Autodesk Fusion 360 part; units mm, degrees
(part 13 of 25)
  arc A2546 (13.97, 2.3813) -> (13.97, 2.6987) centre (13.97, 2.54) ccw
  arc A2547 (73.405, 4.2862) -> (73.405, 4.6038) centre (73.405, 4.445) ccw
  arc A2548 (40.64, 5.2388) -> (40.64, 4.9212) centre (40.64, 5.08) ccw
  arc A2549 (38.1, 5.2388) -> (38.1, 4.9212) centre (38.1, 5.08) ccw
  arc A2550 (41.9535, 4.9212) -> (41.9535, 5.2388) centre (41.9535, 5.08) ccw
  arc A2551 (3.9718, 4.9212) -> (3.9718, 5.2388) centre (3.9718, 5.08) ccw
  arc A2552 (34.3335, 4.9212) -> (34.3335, 5.2388) centre (34.3335, 5.08) ccw
  arc A2553 (31.7935, 4.9212) -> (31.7935, 5.2388) centre (31.7935, 5.08) ccw
  arc A2554 (39.8168, 4.9212) -> (39.8168, 5.2388) centre (39.8168, 5.08) ccw
  arc A2555 (82.5144, 3.3338) -> (82.5144, 3.0163) centre (82.5144, 3.1751) ccw
  line L888 (34.2465, 5.08) -> (34.3335, 5.08)
  line L889 (41.4632, 5.08) -> (41.9535, 5.08)
  arc A2556 (84.2253, 1.7463) -> (84.2253, 2.0638) centre (84.2253, 1.9051) ccw
  arc A2557 (5.8036, 2.6987) -> (5.8036, 2.3813) centre (5.8036, 2.54) ccw
  arc A2558 (15.0528, 5.2388) -> (15.0528, 4.9212) centre (15.0528, 5.08) ccw
  arc A2559 (80.0301, 1.1113) -> (80.0301, 1.4287) centre (80.0301, 1.27) ccw
  arc A2560 (13.97, 3.6513) -> (13.97, 3.9688) centre (13.97, 3.81) ccw
  arc A2561 (84.2253, 3.6513) -> (84.2253, 3.9688) centre (84.2253, 3.81) ccw
  arc A2562 (6.477, 3.9688) -> (6.477, 3.6513) centre (6.477, 3.81) ccw
  arc A2563 (12.8872, 4.9212) -> (12.8872, 5.2388) centre (12.8872, 5.08) ccw
  arc A2564 (13.97, 2.6987) -> (13.97, 2.3813) centre (13.97, 2.54) ccw
  arc A2565 (37.2768, 4.9212) -> (37.2768, 5.2388) centre (37.2768, 5.08) ccw
  arc A2566 (72.7411, 1.7463) -> (72.7411, 2.0638) centre (72.7411, 1.9051) ccw
  arc A2567 (32.964, 1.1113) -> (32.964, 1.4287) centre (32.964, 1.27) ccw
  arc A2568 (68.4207, 3.9688) -> (68.4207, 3.6513) centre (68.4207, 3.81) ccw
  arc A2569 (57.0166, 33.4949) -> (56.6991, 33.4949) centre (56.8578, 33.4949) ccw
  arc A2570 (84.2253, 3.0163) -> (84.2253, 3.3338) centre (84.2253, 3.1751) ccw
  arc A2571 (56.9702, 19.5673) -> (56.7456, 19.3428) centre (56.8579, 19.455) ccw
  arc A2572 (32.964, 2.3813) -> (32.964, 2.6987) centre (32.964, 2.54) ccw
  arc A2573 (56.7962, 33.6406) -> (57.0895, 33.5191) centre (56.9428, 33.5799) ccw
  arc A2574 (40.64, 5.8738) -> (40.64, 5.5562) centre (40.64, 5.715) ccw
  arc A2575 (62.1865, 5.2388) -> (62.1865, 4.9212) centre (62.1865, 5.08) ccw
  line L890 (54.5665, 5.08) -> (54.6535, 5.08)
  arc A2576 (3.4036, 6.1913) -> (3.4036, 6.5088) centre (3.4036, 6.3501) ccw
  arc A2577 (0.7747, 4.6038) -> (0.7747, 4.2862) centre (0.7747, 4.445) ccw
  arc A2578 (6.731, 6.5088) -> (6.731, 6.1913) centre (6.731, 6.3501) ccw
  arc A2579 (68.5588, 3.3338) -> (68.5588, 3.0163) centre (68.5588, 3.1751) ccw
  arc A2580 (82.2759, 3.9688) -> (82.2759, 3.6513) centre (82.2759, 3.81) ccw
  arc A2581 (52.0265, 5.2388) -> (52.0265, 4.9212) centre (52.0265, 5.08) ccw
  arc A2582 (38.9232, 5.2388) -> (38.9232, 4.9212) centre (38.9232, 5.08) ccw
  arc A2583 (62.2735, 4.9212) -> (62.2735, 5.2388) centre (62.2735, 5.08) ccw
  line L891 (59.6465, 5.08) -> (59.7335, 5.08)
  line L892 (46.9465, 5.08) -> (47.0335, 5.08)
  arc A2584 (84.2253, 4.9212) -> (84.2253, 5.2388) centre (84.2253, 5.08) ccw
  arc A2585 (36.7865, 5.2388) -> (36.7865, 4.9212) centre (36.7865, 5.08) ccw
  line L893 (38.9232, 5.08) -> (39.8168, 5.08)
  line L894 (64.7265, 5.08) -> (64.8135, 5.08)
  line L895 (67.2665, 5.08) -> (67.3535, 5.08)
  arc A2586 (15.6337, 5.8738) -> (15.6337, 5.5562) centre (15.6337, 5.715) ccw
  arc A2587 (40.64, 5.5562) -> (40.64, 5.8738) centre (40.64, 5.715) ccw
  arc A2588 (74.7818, 5.8738) -> (74.7818, 5.5562) centre (74.7818, 5.715) ccw
  arc A2589 (3.4036, 5.5562) -> (3.4036, 5.8738) centre (3.4036, 5.715) ccw
  arc A2590 (67.3535, 4.9212) -> (67.3535, 5.2388) centre (67.3535, 5.08) ccw
  arc A2591 (52.1135, 4.9212) -> (52.1135, 5.2388) centre (52.1135, 5.08) ccw
  arc A2592 (54.6535, 4.9212) -> (54.6535, 5.2388) centre (54.6535, 5.08) ccw
  arc A2593 (12.6114, 4.2862) -> (12.6114, 4.6038) centre (12.6114, 4.445) ccw
  arc A2594 (15.3286, 4.6038) -> (15.3286, 4.2862) centre (15.3286, 4.445) ccw
  arc A2595 (38.1, 4.9212) -> (38.1, 5.2388) centre (38.1, 5.08) ccw
  arc A2596 (64.7265, 5.2388) -> (64.7265, 4.9212) centre (64.7265, 5.08) ccw
  arc A2597 (32.964, 3.0163) -> (32.964, 3.3338) centre (32.964, 3.1751) ccw
  arc A2598 (0.7747, 5.2388) -> (0.7747, 4.9212) centre (0.7747, 5.08) ccw
  arc A2599 (79.9074, 4.2862) -> (79.9074, 4.6038) centre (79.9074, 4.445) ccw
  arc A2600 (44.4065, 5.2388) -> (44.4065, 4.9212) centre (44.4065, 5.08) ccw
  arc A2601 (57.1065, 5.2388) -> (57.1065, 4.9212) centre (57.1065, 5.08) ccw
  arc A2602 (12.3063, 5.5562) -> (12.3063, 5.8738) centre (12.3063, 5.715) ccw
  arc A2603 (3.7214, 4.2862) -> (3.7214, 4.6038) centre (3.7214, 4.445) ccw
  arc A2604 (64.8135, 4.9212) -> (64.8135, 5.2388) centre (64.8135, 5.08) ccw
  arc A2605 (84.2253, 5.5562) -> (84.2253, 5.8738) centre (84.2253, 5.715) ccw
  arc A2606 (34.2465, 5.2388) -> (34.2465, 4.9212) centre (34.2465, 5.08) ccw
  arc A2607 (44.4935, 4.9212) -> (44.4935, 5.2388) centre (44.4935, 5.08) ccw
  line L896 (36.7865, 5.08) -> (37.2768, 5.08)
  arc A2608 (73.7116, 5.5562) -> (73.7116, 5.8738) centre (73.7116, 5.715) ccw
  arc A2609 (84.2253, 4.2862) -> (84.2253, 4.6038) centre (84.2253, 4.445) ccw
  arc A2610 (0.7747, 3.9688) -> (0.7747, 3.6513) centre (0.7747, 3.81) ccw
  arc A2611 (3.6576, 3.6513) -> (3.6576, 3.9688) centre (3.6576, 3.81) ccw
  arc A2612 (49.4865, 5.2388) -> (49.4865, 4.9212) centre (49.4865, 5.08) ccw
  arc A2613 (75.0884, 4.6038) -> (75.0884, 4.2862) centre (75.0884, 4.445) ccw
  arc A2614 (59.7335, 4.9212) -> (59.7335, 5.2388) centre (59.7335, 5.08) ccw
  arc A2615 (69.8065, 5.2388) -> (69.8065, 4.9212) centre (69.8065, 5.08) ccw
  arc A2616 (6.1628, 5.2388) -> (6.1628, 4.9212) centre (6.1628, 5.08) ccw
  arc A2617 (81.5908, 4.6038) -> (81.5908, 4.2862) centre (81.5908, 4.445) ccw
  arc A2618 (29.4986, 5.5562) -> (29.4986, 5.8738) centre (29.4986, 5.715) ccw
  arc A2619 (38.1, 5.8738) -> (38.1, 5.5562) centre (38.1, 5.715) ccw
  arc A2620 (44.4935, 7.4612) -> (44.4935, 7.7788) centre (44.4935, 7.62) ccw
  arc A2621 (40.64, 6.8262) -> (40.64, 7.1438) centre (40.64, 6.985) ccw
  arc A2622 (82.1916, 6.5088) -> (82.1916, 6.1913) centre (82.1916, 6.3501) ccw
  arc A2623 (57.1935, 4.9212) -> (57.1935, 5.2388) centre (57.1935, 5.08) ccw
  arc A2624 (80.214, 5.5562) -> (80.214, 5.8738) centre (80.214, 5.715) ccw
  arc A2625 (31.7935, 7.4612) -> (31.7935, 7.7788) centre (31.7935, 7.62) ccw
  arc A2626 (34.2465, 7.7788) -> (34.2465, 7.4612) centre (34.2465, 7.62) ccw
  arc A2627 (46.9465, 5.2388) -> (46.9465, 4.9212) centre (46.9465, 5.08) ccw
  arc A2628 (41.4632, 7.7788) -> (41.4632, 7.4612) centre (41.4632, 7.62) ccw
  arc A2629 (54.5665, 5.2388) -> (54.5665, 4.9212) centre (54.5665, 5.08) ccw
  arc A2630 (3.9972, 7.4612) -> (3.9972, 7.7788) centre (3.9972, 7.62) ccw
  arc A2631 (40.64, 7.1438) -> (40.64, 6.8262) centre (40.64, 6.985) ccw
  arc A2632 (12.3063, 6.1913) -> (12.3063, 6.5088) centre (12.3063, 6.3501) ccw
  arc A2633 (15.6337, 6.5088) -> (15.6337, 6.1913) centre (15.6337, 6.3501) ccw
  arc A2634 (49.5735, 4.9212) -> (49.5735, 5.2388) centre (49.5735, 5.08) ccw
  arc A2635 (70.7429, 6.8262) -> (70.7429, 7.1438) centre (70.7429, 6.985) ccw
  arc A2636 (0.7747, 7.7788) -> (0.7747, 7.4612) centre (0.7747, 7.62) ccw
  line L897 (57.1065, 5.08) -> (57.1935, 5.08)
  line L898 (62.1865, 5.08) -> (62.2735, 5.08)
  arc A2637 (0.7747, 6.5088) -> (0.7747, 6.1913) centre (0.7747, 6.3501) ccw
  arc A2638 (67.2665, 5.2388) -> (67.2665, 4.9212) centre (67.2665, 5.08) ccw
  arc A2639 (38.1, 7.7788) -> (38.1, 7.4612) centre (38.1, 7.62) ccw
  arc A2640 (70.2277, 7.1438) -> (70.2277, 6.8262) centre (70.2277, 6.985) ccw
  arc A2641 (34.3335, 7.4612) -> (34.3335, 7.7788) centre (34.3335, 7.62) ccw
  arc A2642 (79.3067, 6.1913) -> (79.3067, 6.5088) centre (79.3067, 6.3501) ccw
  line L899 (38.1, 6.35) -> (40.64, 6.35)
  arc A2643 (15.6337, 7.1438) -> (15.6337, 6.8262) centre (15.6337, 6.985) ccw
  arc A2644 (38.1, 5.5562) -> (38.1, 5.8738) centre (38.1, 5.715) ccw
  arc A2645 (0.7747, 5.8738) -> (0.7747, 5.5562) centre (0.7747, 5.715) ccw
  arc A2646 (59.6465, 5.2388) -> (59.6465, 4.9212) centre (59.6465, 5.08) ccw
  arc A2647 (75.6891, 6.5088) -> (75.6891, 6.1913) centre (75.6891, 6.3501) ccw
  arc A2648 (40.64, 7.7788) -> (40.64, 7.4612) centre (40.64, 7.62) ccw
  arc A2649 (6.731, 5.8738) -> (6.731, 5.5562) centre (6.731, 5.715) ccw
  line L900 (46.9465, 7.62) -> (47.0335, 7.62)
  arc A2650 (40.64, 6.1913) -> (40.64, 6.5088) centre (40.64, 6.3501) ccw
  arc A2651 (47.0335, 7.4612) -> (47.0335, 7.7788) centre (47.0335, 7.62) ccw
  arc A2652 (6.1374, 7.7788) -> (6.1374, 7.4612) centre (6.1374, 7.62) ccw
  arc A2653 (3.4036, 6.8262) -> (3.4036, 7.1438) centre (3.4036, 6.985) ccw
  arc A2654 (38.1, 6.8262) -> (38.1, 7.1438) centre (38.1, 6.985) ccw
  arc A2655 (0.7747, 7.1438) -> (0.7747, 6.8262) centre (0.7747, 6.985) ccw
  arc A2656 (11.317, 7.4612) -> (11.317, 7.7788) centre (11.317, 7.62) ccw
  arc A2657 (81.2842, 5.8738) -> (81.2842, 5.5562) centre (81.2842, 5.715) ccw
  arc A2658 (28.8636, 6.1913) -> (28.8636, 6.5088) centre (28.8636, 6.3501) ccw
  arc A2659 (70.2277, 5.8738) -> (70.2277, 5.5562) centre (70.2277, 5.715) ccw
  line L901 (44.4065, 5.08) -> (44.4935, 5.08)
  arc A2660 (38.1, 7.1438) -> (38.1, 6.8262) centre (38.1, 6.985) ccw
  arc A2661 (41.9535, 7.4612) -> (41.9535, 7.7788) centre (41.9535, 7.62) ccw
  line L902 (49.4865, 5.08) -> (49.5735, 5.08)
  arc A2662 (47.0335, 4.9212) -> (47.0335, 5.2388) centre (47.0335, 5.08) ccw
  line L903 (52.0265, 5.08) -> (52.1135, 5.08)
  arc A2663 (11.952, 6.8262) -> (11.952, 7.1438) centre (11.952, 6.985) ccw
  arc A2664 (59.6465, 7.7788) -> (59.6465, 7.4612) centre (59.6465, 7.62) ccw
  arc A2665 (84.2253, 8.0963) -> (84.2253, 8.4138) centre (84.2253, 8.2551) ccw
  arc A2666 (54.6535, 7.4612) -> (54.6535, 7.7788) centre (54.6535, 7.62) ccw
  arc A2667 (40.64, 7.4612) -> (40.64, 7.7788) centre (40.64, 7.62) ccw
  line L904 (49.4865, 7.62) -> (49.5735, 7.62)
  line L905 (62.1865, 7.62) -> (62.2735, 7.62)
  arc A2668 (26.3236, 8.7313) -> (26.3236, 9.0488) centre (26.3236, 8.89) ccw
  arc A2669 (82.983, 8.4138) -> (82.983, 8.0963) centre (82.983, 8.2551) ccw
  arc A2670 (37.2768, 7.4612) -> (37.2768, 7.7788) centre (37.2768, 7.62) ccw
  line L906 (34.2465, 7.62) -> (34.3335, 7.62)
  arc A2671 (44.4065, 7.7788) -> (44.4065, 7.4612) centre (44.4065, 7.62) ccw
  arc A2672 (30.8264, 7.7788) -> (30.8264, 7.4612) centre (30.8264, 7.62) ccw
  arc A2673 (84.2253, 6.8262) -> (84.2253, 7.1438) centre (84.2253, 6.985) ccw
  arc A2674 (72.8043, 6.1913) -> (72.8043, 6.5088) centre (72.8043, 6.3501) ccw
  arc A2675 (54.5665, 7.7788) -> (54.5665, 7.4612) centre (54.5665, 7.62) ccw
  arc A2676 (15.0528, 7.7788) -> (15.0528, 7.4612) centre (15.0528, 7.62) ccw
  arc A2677 (27.5936, 7.4612) -> (27.5936, 7.7788) centre (27.5936, 7.62) ccw
  arc A2678 (44.7421, 8.0963) -> (44.7421, 8.4138) centre (44.7421, 8.2551) ccw
  arc A2679 (38.1, 7.4612) -> (38.1, 7.7788) centre (38.1, 7.62) ccw
  arc A2680 (39.8168, 7.4612) -> (39.8168, 7.7788) centre (39.8168, 7.62) ccw
  arc A2681 (52.1135, 7.4612) -> (52.1135, 7.7788) centre (52.1135, 7.62) ccw
  line L907 (69.8065, 7.62) -> (70.1079, 7.62)
  arc A2682 (26.9586, 8.0963) -> (26.9586, 8.4138) centre (26.9586, 8.2551) ccw
  arc A2683 (28.2286, 6.8262) -> (28.2286, 7.1438) centre (28.2286, 6.985) ccw
  arc A2684 (84.2253, 6.1913) -> (84.2253, 6.5088) centre (84.2253, 6.3501) ccw
  arc A2685 (82.4863, 7.1438) -> (82.4863, 6.8262) centre (82.4863, 6.985) ccw
  arc A2686 (13.448, 8.4138) -> (13.448, 8.0963) centre (13.448, 8.2551) ccw
  arc A2687 (70.3453, 6.5088) -> (70.3453, 6.1913) centre (70.3453, 6.3501) ccw
  arc A2688 (46.9465, 7.7788) -> (46.9465, 7.4612) centre (46.9465, 7.62) ccw
  arc A2689 (29.5564, 9.0488) -> (29.5564, 8.7313) centre (29.5564, 8.89) ccw
  arc A2690 (46.6979, 8.4138) -> (46.6979, 8.0963) centre (46.6979, 8.2551) ccw
  arc A2691 (38.1, 6.5088) -> (38.1, 6.1913) centre (38.1, 6.3501) ccw
  arc A2692 (52.0265, 7.7788) -> (52.0265, 7.4612) centre (52.0265, 7.62) ccw
  line L908 (57.1065, 7.62) -> (57.1935, 7.62)
  arc A2693 (59.7335, 7.4612) -> (59.7335, 7.7788) centre (59.7335, 7.62) ccw
  line L909 (64.7265, 7.62) -> (64.8135, 7.62)
  arc A2694 (38.9232, 7.7788) -> (38.9232, 7.4612) centre (38.9232, 7.62) ccw
  arc A2695 (67.2665, 7.7788) -> (67.2665, 7.4612) centre (67.2665, 7.62) ccw
  arc A2696 (69.4729, 8.0963) -> (69.4729, 8.4138) centre (69.4729, 8.2551) ccw
  arc A2697 (36.7865, 7.7788) -> (36.7865, 7.4612) centre (36.7865, 7.62) ccw
  arc A2698 (46.6979, 9.0488) -> (46.6979, 8.7313) centre (46.6979, 8.89) ccw
  arc A2699 (6.731, 7.1438) -> (6.731, 6.8262) centre (6.731, 6.985) ccw
  arc A2700 (68.8379, 8.7313) -> (68.8379, 9.0488) centre (68.8379, 8.89) ccw
  arc A2701 (82.5144, 7.7788) -> (82.5144, 7.4612) centre (82.5144, 7.62) ccw
  arc A2702 (64.8135, 7.4612) -> (64.8135, 7.7788) centre (64.8135, 7.62) ccw
  line L910 (59.6465, 7.62) -> (59.7335, 7.62)
  arc A2703 (4.1275, 8.7313) -> (4.1275, 9.0488) centre (4.1275, 8.89) ccw
  line L911 (52.0265, 7.62) -> (52.1135, 7.62)
  arc A2704 (84.2253, 8.7313) -> (84.2253, 9.0488) centre (84.2253, 8.89) ccw
  arc A2705 (0.7747, 10.3187) -> (0.7747, 10.0013) centre (0.7747, 10.16) ccw
  arc A2706 (30.1914, 8.4138) -> (30.1914, 8.0963) centre (30.1914, 8.2551) ccw
  arc A2707 (28.2864, 10.3187) -> (28.2864, 10.0013) centre (28.2864, 10.16) ccw
  arc A2708 (10.4521, 8.7313) -> (10.4521, 9.0488) centre (10.4521, 8.89) ccw
  arc A2709 (67.3535, 7.4612) -> (67.3535, 7.7788) centre (67.3535, 7.62) ccw
  line L912 (54.5665, 7.62) -> (54.6535, 7.62)
  arc A2710 (64.7265, 7.7788) -> (64.7265, 7.4612) centre (64.7265, 7.62) ccw
  arc A2711 (79.7385, 8.7313) -> (79.7385, 9.0488) centre (79.7385, 8.89) ccw
  arc A2712 (57.1065, 7.7788) -> (57.1065, 7.4612) centre (57.1065, 7.62) ccw
  arc A2713 (3.6263, 10.6363) -> (3.6263, 10.9537) centre (3.6263, 10.795) ccw
  arc A2714 (14.4213, 10.0013) -> (14.4213, 10.3187) centre (14.4213, 10.16) ccw
  arc A2715 (12.813, 9.0488) -> (12.813, 8.7313) centre (12.813, 8.89) ccw
  arc A2716 (12.4079, 10.3187) -> (12.4079, 10.0013) centre (12.4079, 10.16) ccw
  arc A2717 (81.6991, 10.0013) -> (81.6991, 10.3187) centre (81.6991, 10.16) ccw
  arc A2718 (6.0833, 9.6837) -> (6.0833, 9.3663) centre (6.0833, 9.525) ccw
  arc A2719 (84.2253, 7.4612) -> (84.2253, 7.7788) centre (84.2253, 7.62) ccw
  arc A2720 (62.1865, 7.7788) -> (62.1865, 7.4612) centre (62.1865, 7.62) ccw
  arc A2721 (69.8065, 7.7788) -> (69.8065, 7.4612) centre (69.8065, 7.62) ccw
  arc A2722 (46.6979, 10.3187) -> (46.6979, 10.0013) centre (46.6979, 10.16) ccw
  arc A2723 (66.0563, 10.0013) -> (66.0563, 10.3187) centre (66.0563, 10.16) ccw
  arc A2724 (76.313, 10.3187) -> (76.313, 10.0013) centre (76.313, 10.16) ccw
  arc A2725 (6.0833, 9.0488) -> (6.0833, 8.7313) centre (6.0833, 8.89) ccw
  arc A2726 (84.2253, 10.0013) -> (84.2253, 10.3187) centre (84.2253, 10.16) ccw
  arc A2727 (70.372, 10.0013) -> (70.372, 10.3187) centre (70.372, 10.16) ccw
  arc A2728 (83.6549, 10.3187) -> (83.6549, 10.0013) centre (83.6549, 10.16) ccw
  arc A2729 (49.4865, 7.7788) -> (49.4865, 7.4612) centre (49.4865, 7.62) ccw
  arc A2730 (4.1275, 10.0013) -> (4.1275, 10.3187) centre (4.1275, 10.16) ccw
  arc A2731 (83.5524, 9.0488) -> (83.5524, 8.7313) centre (83.5524, 8.89) ccw
  arc A2732 (6.0833, 8.4138) -> (6.0833, 8.0963) centre (6.0833, 8.2551) ccw
  arc A2733 (71.007, 9.3663) -> (71.007, 9.6837) centre (71.007, 9.525) ccw
  arc A2734 (57.1935, 7.4612) -> (57.1935, 7.7788) centre (57.1935, 7.62) ccw
  arc A2735 (0.7747, 10.9537) -> (0.7747, 10.6363) centre (0.7747, 10.795) ccw
  arc A2736 (10.682, 8.0963) -> (10.682, 8.4138) centre (10.682, 8.2551) ccw
  arc A2737 (25.0536, 10.0013) -> (25.0536, 10.3187) centre (25.0536, 10.16) ccw
  arc A2738 (28.9214, 9.6837) -> (28.9214, 9.3663) centre (28.9214, 9.525) ccw
  arc A2739 (0.7747, 8.4138) -> (0.7747, 8.0963) centre (0.7747, 8.2551) ccw
  arc A2740 (44.7421, 8.7313) -> (44.7421, 9.0488) centre (44.7421, 8.89) ccw
  line L913 (67.2665, 7.62) -> (67.3535, 7.62)
  arc A2741 (4.1275, 8.0963) -> (4.1275, 8.4138) centre (4.1275, 8.2551) ccw
  arc A2742 (16.1095, 10.3187) -> (16.1095, 10.0013) centre (16.1095, 10.16) ccw
  arc A2743 (83.6549, 9.6837) -> (83.6549, 9.3663) centre (83.6549, 9.525) ccw
  arc A2744 (62.2735, 7.4612) -> (62.2735, 7.7788) centre (62.2735, 7.62) ccw
  arc A2745 (71.6038, 9.0488) -> (71.6038, 8.7313) centre (71.6038, 8.89) ccw
  arc A2746 (70.1079, 7.4612) -> (70.1079, 7.7788) centre (70.1079, 7.62) ccw
  arc A2747 (0.7747, 9.0488) -> (0.7747, 8.7313) centre (0.7747, 8.89) ccw
  arc A2748 (49.5735, 7.4612) -> (49.5735, 7.7788) centre (49.5735, 7.62) ccw
  arc A2749 (70.3338, 10.3187) -> (70.3338, 10.0013) centre (70.3338, 10.16) ccw
  arc A2750 (25.6886, 9.3663) -> (25.6886, 9.6837) centre (25.6886, 9.525) ccw
  line L914 (70.3338, 10.16) -> (70.372, 10.16)
  line L915 (70.9688, 9.525) -> (71.007, 9.525)
  arc A2751 (12.4079, 9.6837) -> (12.4079, 9.3663) centre (12.4079, 9.525) ccw
  arc A2752 (84.2253, 9.3663) -> (84.2253, 9.6837) centre (84.2253, 9.525) ccw
  arc A2753 (81.4871, 9.3663) -> (81.4871, 9.6837) centre (81.4871, 9.525) ccw
  arc A2754 (69.102, 11.2713) -> (69.102, 11.5887) centre (69.102, 11.43) ccw
  arc A2755 (81.5916, 11.2713) -> (81.5916, 11.5887) centre (81.5916, 11.43) ccw
  arc A2756 (13.7795, 11.2713) -> (13.7795, 11.5887) centre (13.7795, 11.43) ccw
  arc A2757 (6.0833, 10.3187) -> (6.0833, 10.0013) centre (6.0833, 10.16) ccw
  arc A2758 (0.7747, 9.6837) -> (0.7747, 9.3663) centre (0.7747, 9.525) ccw
  arc A2759 (0.7747, 11.5887) -> (0.7747, 11.2713) centre (0.7747, 11.43) ccw
  arc A2760 (44.7421, 10.6363) -> (44.7421, 10.9537) centre (44.7421, 10.795) ccw
  arc A2761 (77.583, 11.5887) -> (77.583, 11.2713) centre (77.583, 11.43) ccw
  arc A2762 (66.216, 9.3663) -> (66.216, 9.6837) centre (66.216, 9.525) ccw
  arc A2763 (70.9688, 9.6837) -> (70.9688, 9.3663) centre (70.9688, 9.525) ccw
  arc A2764 (16.8945, 11.5887) -> (16.8945, 11.2713) centre (16.8945, 11.43) ccw
  arc A2765 (27.0164, 11.5887) -> (27.0164, 11.2713) centre (27.0164, 11.43) ccw
  arc A2766 (84.2253, 11.2713) -> (84.2253, 11.5887) centre (84.2253, 11.43) ccw
  arc A2767 (44.7421, 10.0013) -> (44.7421, 10.3187) centre (44.7421, 10.16) ccw
  arc A2768 (10.4521, 10.0013) -> (10.4521, 10.3187) centre (10.4521, 10.16) ccw
  arc A2769 (13.8117, 11.9063) -> (13.8117, 12.2238) centre (13.8117, 12.0651) ccw
  arc A2770 (12.178, 12.2238) -> (12.178, 11.9063) centre (12.178, 12.0651) ccw
  arc A2771 (75.678, 9.6837) -> (75.678, 9.3663) centre (75.678, 9.525) ccw
  arc A2772 (10.4521, 9.3663) -> (10.4521, 9.6837) centre (10.4521, 9.525) ccw
  arc A2773 (76.948, 10.9537) -> (76.948, 10.6363) centre (76.948, 10.795) ccw
  arc A2774 (4.1275, 9.3663) -> (4.1275, 9.6837) centre (4.1275, 9.525) ccw
  arc A2775 (24.4185, 10.6363) -> (24.4185, 10.9537) centre (24.4185, 10.795) ccw
  arc A2776 (73.2432, 11.5887) -> (73.2432, 11.2713) centre (73.2432, 11.43) ccw
  arc A2777 (10.047, 11.2713) -> (10.047, 11.5887) centre (10.047, 11.43) ccw
  arc A2778 (13.7863, 10.6363) -> (13.7863, 10.9537) centre (13.7863, 10.795) ccw
  arc A2779 (23.7836, 11.2713) -> (23.7836, 11.5887) centre (23.7836, 11.43) ccw
  arc A2780 (84.2253, 10.6363) -> (84.2253, 10.9537) centre (84.2253, 10.795) ccw
  arc A2781 (73.2361, 8.7313) -> (73.2361, 9.0488) centre (73.2361, 8.89) ccw
  arc A2782 (66.216, 10.6363) -> (66.216, 10.9537) centre (66.216, 10.795) ccw
  arc A2783 (69.737, 10.6363) -> (69.737, 10.9537) centre (69.737, 10.795) ccw
  arc A2784 (3.6195, 11.2713) -> (3.6195, 11.5887) centre (3.6195, 11.43) ccw
  line L916 (69.6988, 10.795) -> (69.737, 10.795)
  arc A2785 (46.6979, 10.9537) -> (46.6979, 10.6363) centre (46.6979, 10.795) ccw
  arc A2786 (12.4079, 10.9537) -> (12.4079, 10.6363) centre (12.4079, 10.795) ccw
  arc A2787 (75.2573, 9.0488) -> (75.2573, 8.7313) centre (75.2573, 8.89) ccw
  arc A2788 (44.7421, 9.3663) -> (44.7421, 9.6837) centre (44.7421, 9.525) ccw
  arc A2789 (46.6979, 9.6837) -> (46.6979, 9.3663) centre (46.6979, 9.525) ccw
  arc A2790 (8.777, 12.5413) -> (8.777, 12.8588) centre (8.777, 12.7001) ccw
  arc A2791 (71.6638, 13.1763) -> (71.6638, 13.4938) centre (71.6638, 13.335) ccw
  arc A2792 (26.3814, 12.2238) -> (26.3814, 11.9063) centre (26.3814, 12.0651) ccw
  arc A2793 (44.7421, 11.2713) -> (44.7421, 11.5887) centre (44.7421, 11.43) ccw
  arc A2794 (27.6514, 10.9537) -> (27.6514, 10.6363) centre (27.6514, 10.795) ccw
  arc A2795 (72.517, 12.8588) -> (72.517, 12.5413) centre (72.517, 12.7001) ccw
  arc A2796 (23.1486, 11.9063) -> (23.1486, 12.2238) centre (23.1486, 12.0651) ccw
  arc A2797 (12.4079, 11.5887) -> (12.4079, 11.2713) centre (12.4079, 11.43) ccw
  arc A2798 (69.6988, 10.9537) -> (69.6988, 10.6363) centre (69.6988, 10.795) ccw
  arc A2799 (6.5845, 10.9537) -> (6.5845, 10.6363) centre (6.5845, 10.795) ccw
  arc A2800 (0.7747, 12.2238) -> (0.7747, 11.9063) centre (0.7747, 12.0651) ccw
  arc A2801 (72.517, 11.2713) -> (72.517, 11.5887) centre (72.517, 11.43) ccw
  arc A2802 (46.6979, 11.5887) -> (46.6979, 11.2713) centre (46.6979, 11.43) ccw
  arc A2803 (46.814, 13.4938) -> (46.814, 13.1763) centre (46.814, 13.335) ccw
  arc A2804 (84.1629, 12.2238) -> (84.1629, 11.9063) centre (84.1629, 12.0651) ccw
  arc A2805 (81.6991, 10.6363) -> (81.6991, 10.9537) centre (81.6991, 10.795) ccw
  arc A2806 (84.2253, 11.9063) -> (84.2253, 12.2238) centre (84.2253, 12.0651) ccw
  arc A2807 (83.7624, 11.5887) -> (83.7624, 11.2713) centre (83.7624, 11.43) ccw
  arc A2808 (16.7445, 10.9537) -> (16.7445, 10.6363) centre (16.7445, 10.795) ccw
  arc A2809 (0.7747, 12.8588) -> (0.7747, 12.5413) centre (0.7747, 12.7001) ccw
  arc A2810 (69.963, 13.4938) -> (69.963, 13.1763) centre (69.963, 13.335) ccw
  arc A2811 (6.5913, 11.5887) -> (6.5913, 11.2713) centre (6.5913, 11.43) ccw
  arc A2812 (72.517, 12.2238) -> (72.517, 11.9063) centre (72.517, 12.0651) ccw
  arc A2813 (10.4521, 10.6363) -> (10.4521, 10.9537) centre (10.4521, 10.795) ccw
  arc A2814 (9.412, 11.9063) -> (9.412, 12.2238) centre (9.412, 12.0651) ccw
  arc A2815 (15.5667, 13.1763) -> (15.5667, 13.4938) centre (15.5667, 13.335) ccw
  arc A2816 (78.218, 12.2238) -> (78.218, 11.9063) centre (78.218, 12.0651) ccw
  arc A2817 (22.5714, 12.2238) -> (22.5714, 11.9063) centre (22.5714, 12.0651) ccw
  arc A2818 (5.9241, 12.8588) -> (5.9241, 12.5413) centre (5.9241, 12.7001) ccw
  arc A2819 (68.467, 11.9063) -> (68.467, 12.2238) centre (68.467, 12.0651) ccw
  line L917 (71.233, 12.065) -> (71.2851, 12.065)
  arc A2820 (74.817, 11.2713) -> (74.817, 11.5887) centre (74.817, 11.43) ccw
  arc A2821 (25.1114, 13.4938) -> (25.1114, 13.1763) centre (25.1114, 13.335) ccw
  arc A2822 (6.5591, 12.2238) -> (6.5591, 11.9063) centre (6.5591, 12.0651) ccw
  arc A2823 (44.7421, 12.5413) -> (44.7421, 12.8588) centre (44.7421, 12.7001) ccw
  arc A2824 (72.517, 11.5887) -> (72.517, 11.2713) centre (72.517, 11.43) ccw
  arc A2825 (84.1629, 12.8588) -> (84.1629, 12.5413) centre (84.1629, 12.7001) ccw
  arc A2826 (44.626, 13.1763) -> (44.626, 13.4938) centre (44.626, 13.335) ccw
  arc A2827 (48.782, 13.1763) -> (48.782, 13.4938) centre (48.782, 13.335) ccw
  arc A2828 (0.7747, 13.4938) -> (0.7747, 13.1763) centre (0.7747, 13.335) ccw
  arc A2829 (10.908, 13.4938) -> (10.908, 13.1763) centre (10.908, 13.335) ccw
  arc A2830 (78.853, 12.8588) -> (78.853, 12.5413) centre (78.853, 12.7001) ccw
  arc A2831 (83.6549, 10.9537) -> (83.6549, 10.6363) centre (83.6549, 10.795) ccw
  arc A2832 (73.7489, 12.8588) -> (73.7489, 12.5413) centre (73.7489, 12.7001) ccw
  arc A2833 (3.6517, 11.9063) -> (3.6517, 12.2238) centre (3.6517, 12.0651) ccw
  arc A2834 (20.4787, 38.1) -> (20.1612, 38.1) centre (20.32, 38.1) ccw
  line L918 (20.32, 36.8681) -> (20.32, 38.1)
  arc A2835 (18.9206, 36.918) -> (19.1073, 37.1748) centre (19.014, 37.0464) ccw
  line L919 (20.32, 38.1) -> (20.32, 36.8681)
  arc A2836 (18.8322, 37.4097) -> (18.6077, 37.1852) centre (18.72, 37.2975) ccw
  arc A2837 (21.8762, 37.0319) -> (21.6896, 37.2888) centre (21.7829, 37.1604) ccw
  line L920 (18.518, 37.6271) -> (18.606, 37.4543)
  arc A2838 (21.5327, 37.1748) -> (21.7194, 36.918) centre (21.6261, 37.0464) ccw
  arc A2839 (21.0525, 37.0249) -> (21.1022, 36.7113) centre (21.0773, 36.8681) ccw
  line L921 (18.606, 37.4543) -> (18.72, 37.2975)
  arc A2840 (20.32, 38.2587) -> (20.32, 37.9412) centre (20.32, 38.0999) ccw
  arc A2841 (19.086, 37.1878) -> (18.9419, 36.9049) centre (19.014, 37.0464) ccw
  line L922 (20.32, 38.1) -> (18.4277, 38.1)
  arc A2842 (21.0774, 36.7094) -> (21.0774, 37.0268) centre (21.0774, 36.8681) ccw
  arc A2843 (18.7448, 37.0481) -> (18.9693, 37.2726) centre (18.8571, 37.1603) ccw
  arc A2844 (21.6981, 36.9049) -> (21.554, 37.1878) centre (21.6261, 37.0464) ccw
  arc A2845 (18.7344, 37.5477) -> (18.4776, 37.361) centre (18.606, 37.4543) ccw
  arc A2846 (21.3812, 37.0998) -> (21.5254, 36.8169) centre (21.4533, 36.9583) ccw
  line L923 (18.458, 37.8115) -> (18.518, 37.6271)
  arc A2847 (18.3012, 37.7867) -> (18.6148, 37.8364) centre (18.458, 37.8115) ccw
  line L924 (21.0774, 36.8681) -> (21.2689, 36.8984)
  arc A2848 (19.5378, 36.7113) -> (19.5875, 37.0249) centre (19.5627, 36.8681) ccw
  arc A2849 (18.367, 37.5781) -> (18.6689, 37.6762) centre (18.5179, 37.6272) ccw
  arc A2850 (18.6594, 37.6992) -> (18.3765, 37.555) centre (18.5179, 37.6271) ccw
  arc A2851 (20.1612, 38.1) -> (20.4787, 38.1) centre (20.32, 38.1) ccw
  arc A2852 (19.5626, 37.0268) -> (19.5626, 36.7094) centre (19.5626, 36.8681) ccw
  arc A2853 (18.269, 38.003) -> (18.5865, 38.003) centre (18.4277, 38.003) ccw
  arc A2854 (18.4277, 38.2588) -> (18.4277, 37.9413) centre (18.4277, 38.1) ccw
  line L925 (21.2689, 36.8984) -> (21.4533, 36.9584)
  line L926 (19.3711, 36.8984) -> (19.5626, 36.8681)
  arc A2855 (20.1612, 36.8681) -> (20.4787, 36.8681) centre (20.32, 36.8681) ccw
  arc A2856 (19.2358, 37.1093) -> (19.1377, 36.8074) centre (19.1867, 36.9583) ccw
  arc A2857 (18.5865, 38.1) -> (18.269, 38.1) centre (18.4277, 38.1) ccw
  arc A2858 (20.4787, 38.1) -> (20.1612, 38.1) centre (20.32, 38.1) ccw
  arc A2859 (19.1146, 36.8169) -> (19.2588, 37.0998) centre (19.1867, 36.9584) ccw
  arc A2860 (21.5406, 39.3753) -> (21.3965, 39.0924) centre (21.4686, 39.2339) ccw
  arc A2861 (20.32, 37.9413) -> (20.32, 38.2588) centre (20.32, 38.1) ccw
  arc A2862 (20.32, 37.9412) -> (20.32, 38.2587) centre (20.32, 38.0999) ccw
  line L927 (18.4277, 38.1) -> (18.4277, 38.003)
  arc A2863 (18.5845, 38.0279) -> (18.2709, 37.9782) centre (18.4277, 38.0031) ccw
  line L928 (20.32, 36.8681) -> (21.0774, 36.8681)
  arc A2864 (18.4277, 38.2587) -> (18.4277, 37.9412) centre (18.4277, 38.0999) ccw
  arc A2865 (21.5023, 36.8074) -> (21.4042, 37.1093) centre (21.4533, 36.9583) ccw
  line L929 (18.4277, 38.1) -> (20.32, 38.1)
  arc A2866 (18.9504, 37.2888) -> (18.7638, 37.0319) centre (18.8571, 37.1604) ccw
  arc A2867 (19.3221, 36.7475) -> (19.4202, 37.0494) centre (19.3712, 36.8984) ccw
  arc A2868 (20.32, 36.7093) -> (20.32, 37.0268) centre (20.32, 36.8681) ccw
  line L930 (19.1867, 36.9584) -> (19.3711, 36.8984)
  line L931 (19.5626, 36.8681) -> (20.32, 36.8681)
  arc A2869 (18.5915, 37.2042) -> (18.8484, 37.3908) centre (18.72, 37.2975) ccw
  arc A2870 (20.1613, 36.8681) -> (20.4788, 36.8681) centre (20.3201, 36.8681) ccw
  arc A2871 (20.4788, 38.1) -> (20.1613, 38.1) centre (20.3201, 38.1) ccw
  arc A2872 (21.2198, 37.0494) -> (21.3179, 36.7475) centre (21.2688, 36.8984) ccw
  line L932 (21.6261, 37.0464) -> (21.7829, 37.1604)
  line L933 (18.4277, 38.003) -> (18.458, 37.8115)
  arc A2873 (20.32, 37.9412) -> (20.32, 38.2587) centre (20.32, 38.0999) ccw
  line L934 (18.72, 37.2975) -> (18.8571, 37.1604)
  arc A2874 (18.4645, 37.3823) -> (18.7474, 37.5264) centre (18.6059, 37.4544) ccw
  arc A2875 (18.609, 37.8606) -> (18.3071, 37.7625) centre (18.4581, 37.8116) ccw
  arc A2876 (19.396, 37.0552) -> (19.3463, 36.7416) centre (19.3712, 36.8984) ccw
  line L935 (19.0139, 37.0464) -> (19.1867, 36.9584)
  line L936 (18.8571, 37.1604) -> (19.0139, 37.0464)
  arc A2877 (20.32, 37.0268) -> (20.32, 36.7094) centre (20.32, 36.8681) ccw
  arc A2878 (22.0252, 37.8364) -> (22.3388, 37.7867) centre (22.182, 37.8115) ccw
  arc A2879 (20.32, 38.2588) -> (20.32, 37.9413) centre (20.32, 38.1) ccw
  arc A2880 (21.554, 39.0122) -> (21.6981, 39.2951) centre (21.6261, 39.1536) ccw
  line L937 (21.8221, 39.3803) -> (22.1039, 39.6621)
  arc A2881 (22.031, 38.3394) -> (22.3329, 38.4375) centre (22.1819, 38.3884) ccw
  arc A2882 (22.0535, 38.1) -> (22.371, 38.1) centre (22.2123, 38.1) ccw
  arc A2883 (21.7194, 39.282) -> (21.5327, 39.0252) centre (21.626, 39.1536) ccw
  arc A2884 (21.4078, 39.3805) -> (21.5293, 39.0872) centre (21.4686, 39.2339) ccw
  line L938 (20.32, 38.1) -> (22.2123, 38.1)
  arc A2885 (22.3329, 37.7625) -> (22.031, 37.8606) centre (22.1819, 37.8116) ccw
  line L939 (22.2123, 38.1) -> (20.32, 38.1)
  arc A2886 (15.0857, 36.2682) -> (14.7923, 36.1467) centre (14.939, 36.2075) ccw
  arc A2887 (21.6896, 38.9112) -> (21.8762, 39.1681) centre (21.7829, 39.0397) ccw
  arc A2888 (22.3691, 37.9782) -> (22.0555, 38.0279) centre (22.2123, 38.0031) ccw
  line L940 (22.182, 37.8115) -> (22.2123, 38.003)
  line L941 (21.7829, 37.1604) -> (21.92, 37.2975)
  line L942 (22.2123, 38.197) -> (22.182, 38.3885)
  arc A2889 (20.4788, 38.1) -> (20.1613, 38.1) centre (20.3201, 38.1) ccw
  arc A2890 (22.0555, 38.1721) -> (22.3691, 38.2218) centre (22.2123, 38.197) ccw
  arc A2891 (25.5945, 39.5034) -> (25.5945, 39.8209) centre (25.5945, 39.6622) ccw
  line L943 (22.2123, 38.003) -> (22.2123, 38.1)
  line L944 (25.9539, 39.811) -> (26.5671, 40.4241)
  line L945 (22.2123, 38.1) -> (22.2123, 38.197)
  line L946 (21.6261, 39.1536) -> (21.4685, 39.2339)
  arc A2892 (25.5338, 39.8088) -> (25.6553, 39.5154) centre (25.5946, 39.6621) ccw
  arc A2893 (22.2123, 37.9412) -> (22.2123, 38.2587) centre (22.2123, 38.0999) ccw
  arc A2894 (22.0323, 37.1852) -> (21.8078, 37.4097) centre (21.92, 37.2975) ccw
  arc A2895 (20.1613, 38.1) -> (20.4788, 38.1) centre (20.3201, 38.1) ccw
  arc A2896 (22.2161, 39.5498) -> (21.9916, 39.7744) centre (22.1039, 39.6621) ccw
  line L947 (22.182, 38.3885) -> (22.122, 38.5729)
  line L948 (21.7829, 39.0396) -> (21.6261, 39.1536)
  line L949 (22.034, 37.4543) -> (22.122, 37.6271)
  line L950 (22.034, 38.7457) -> (21.92, 38.9025)
  arc A2897 (22.1039, 39.8209) -> (22.1039, 39.5034) centre (22.1039, 39.6622) ccw
  arc A2898 (21.8078, 38.7903) -> (22.0323, 39.0148) centre (21.92, 38.9026) ccw
  arc A2899 (21.8952, 39.1519) -> (21.6707, 38.9274) centre (21.783, 39.0396) ccw
  arc A2900 (22.2123, 37.9413) -> (22.2123, 38.2588) centre (22.2123, 38.1) ccw
  line L951 (21.92, 37.2975) -> (22.034, 37.4543)
  arc A2901 (22.0485, 38.9958) -> (21.7916, 38.8092) centre (21.92, 38.9025) ccw
  arc A2902 (21.7098, 39.4926) -> (21.9343, 39.2681) centre (21.822, 39.3803) ccw
  arc A2903 (22.1624, 37.361) -> (21.9056, 37.5477) centre (22.034, 37.4543) ccw
  arc A2904 (22.3388, 38.4133) -> (22.0252, 38.3636) centre (22.182, 38.3884) ccw
  arc A2905 (26.6793, 40.3118) -> (26.4548, 40.5364) centre (26.5671, 40.4241) ccw
  arc A2906 (21.6707, 37.2726) -> (21.8952, 37.0481) centre (21.783, 37.1603) ccw
  arc A2907 (22.371, 38.1) -> (22.0535, 38.1) centre (22.2123, 38.1) ccw
  line L952 (22.1039, 39.6621) -> (25.5945, 39.6621)
  line L953 (22.122, 37.6271) -> (22.182, 37.8115)
  arc A2908 (21.9056, 38.6523) -> (22.1624, 38.839) centre (22.034, 38.7457) ccw
  arc A2909 (21.8828, 39.2336) -> (21.7613, 39.527) centre (21.8221, 39.3803) ccw
  arc A2910 (21.9711, 37.6762) -> (22.273, 37.5781) centre (22.1221, 37.6272) ccw
  line L954 (25.5945, 39.6621) -> (25.9539, 39.811)
  arc A2911 (26.0147, 39.6643) -> (25.8932, 39.9576) centre (25.954, 39.8109) ccw
  arc A2912 (21.7916, 37.3908) -> (22.0485, 37.2042) centre (21.92, 37.2975) ccw
  line L955 (22.122, 38.5729) -> (22.034, 38.7457)
  line L956 (21.4685, 39.2339) -> (21.8221, 39.3803)
  arc A2913 (22.273, 38.6219) -> (21.9711, 38.5238) centre (22.1221, 38.5729) ccw
  arc A2914 (21.8926, 37.5264) -> (22.1755, 37.3823) centre (22.0341, 37.4544) ccw
  arc A2915 (20.32, 38.2587) -> (20.32, 37.9412) centre (20.32, 38.0999) ccw
  arc A2916 (22.2635, 37.555) -> (21.9806, 37.6992) centre (22.1221, 37.6271) ccw
  arc A2917 (22.0535, 38.003) -> (22.371, 38.003) centre (22.2123, 38.003) ccw
  arc A2918 (22.371, 38.197) -> (22.0535, 38.197) centre (22.2123, 38.197) ccw
  arc A2919 (22.1755, 38.8177) -> (21.8926, 38.6736) centre (22.0341, 38.7457) ccw
  arc A2920 (21.9806, 38.5008) -> (22.2635, 38.645) centre (22.1221, 38.5729) ccw
  line L957 (21.92, 38.9025) -> (21.7829, 39.0396)
  arc A2921 (37.4455, 43.2371) -> (37.4455, 43.5546) centre (37.4455, 43.3959) ccw
  arc A2922 (25.8417, 39.9232) -> (26.0662, 39.6987) centre (25.954, 39.811) ccw
  arc A2923 (38.1571, 41.2945) -> (38.4746, 41.2945) centre (38.3158, 41.2945) ccw
  arc A2924 (36.1023, 40.3118) -> (36.3268, 40.5364) centre (36.2145, 40.4241) ccw
  arc A2925 (27.1732, 40.5364) -> (27.3977, 40.3118) centre (27.2855, 40.4241) ccw
  arc A2926 (15.2717, 35.7874) -> (14.9542, 35.7874) centre (15.113, 35.7874) ccw
  arc A2927 (11.6574, 39.0842) -> (11.6574, 39.4017) centre (11.6574, 39.243) ccw
  arc A2928 (37.3332, 40.5364) -> (37.5577, 40.3118) centre (37.4455, 40.4241) ccw
  arc A2929 (36.2145, 43.5546) -> (36.2145, 43.2371) centre (36.2145, 43.3959) ccw
  arc A2930 (35.5029, 42.5255) -> (35.1854, 42.5255) centre (35.3441, 42.5255) ccw
  arc A2931 (12.2867, 38.6352) -> (12.5112, 38.8597) centre (12.399, 38.7475) ccw
  arc A2932 (4.3767, 40.6443) -> (4.1522, 40.4197) centre (4.2645, 40.532) ccw
  line L958 (15.113, 35.7874) -> (14.939, 36.2075)
  arc A2933 (14.7297, 36.6412) -> (14.5052, 36.4167) centre (14.6175, 36.529) ccw
  arc A2934 (14.5052, 36.4167) -> (14.7297, 36.6412) centre (14.6175, 36.529) ccw
  line L959 (37.4455, 40.4241) -> (38.3159, 41.2945)
  arc A2935 (15.5271, 34.9122) -> (15.2337, 34.7907) centre (15.3804, 34.8514) ccw
  arc A2936 (12.5112, 38.8597) -> (12.2867, 38.6352) centre (12.399, 38.7475) ccw
  line L960 (35.3441, 42.5255) -> (35.3441, 41.2945)
  arc A2937 (5.5534, 39.4017) -> (5.5534, 39.0842) centre (5.5534, 39.243) ccw
  arc A2938 (11.7181, 39.3897) -> (11.5966, 39.0963) centre (11.6573, 39.243) ccw
  line L961 (36.2145, 43.3959) -> (35.3441, 42.5255)
  arc A2939 (15.7924, 34.2399) -> (15.4749, 34.2399) centre (15.6337, 34.2399) ccw
  arc A2940 (35.2318, 42.6377) -> (35.4564, 42.4132) centre (35.3441, 42.5255) ccw
  line L962 (14.939, 36.2075) -> (14.6175, 36.529)
  line L963 (14.6175, 36.529) -> (12.399, 38.7475)
  line L964 (37.4455, 43.3959) -> (36.2145, 43.3959)
  line L965 (38.3159, 42.5255) -> (37.4455, 43.3959)
  arc A2941 (35.4564, 41.4068) -> (35.2318, 41.1823) centre (35.3441, 41.2946) ccw
  arc A2942 (28.2682, 41.1823) -> (28.0436, 41.4068) centre (28.1559, 41.2946) ccw
  line L966 (38.3159, 41.2945) -> (38.3159, 42.5255)
  arc A2943 (38.4282, 41.1823) -> (38.2036, 41.4068) centre (38.3159, 41.2945) ccw
  line L967 (12.399, 38.7475) -> (12.0775, 39.069)
  arc A2944 (14.8267, 36.0952) -> (15.0512, 36.3197) centre (14.939, 36.2075) ccw
  arc A2945 (27.2855, 40.2654) -> (27.2855, 40.5829) centre (27.2855, 40.4241) ccw
  line L968 (5.5534, 39.243) -> (4.2644, 40.532)
  arc A2946 (15.4749, 33.5781) -> (15.7924, 33.5781) centre (15.6337, 33.5781) ccw
  arc A2947 (15.487, 34.1792) -> (15.7804, 34.3007) centre (15.6337, 34.24) ccw
  line L969 (15.113, 35.1188) -> (15.113, 35.7874)
  line L970 (11.6574, 39.243) -> (5.5534, 39.243)
  arc A2948 (37.4455, 40.2654) -> (37.4455, 40.5829) centre (37.4455, 40.4241) ccw
  line L971 (12.0775, 39.069) -> (11.6574, 39.243)
  line L972 (15.3804, 34.8514) -> (15.113, 35.1188)
  arc A2949 (35.1854, 41.2945) -> (35.5029, 41.2945) centre (35.3441, 41.2945) ccw
  line L973 (15.6337, 33.5781) -> (15.6337, 34.2399)
  line L974 (27.2855, 40.4241) -> (28.1559, 41.2945)
  arc A2950 (38.4746, 42.5255) -> (38.1571, 42.5255) centre (38.3158, 42.5255) ccw
  arc A2951 (5.4412, 39.1307) -> (5.6657, 39.3553) centre (5.5535, 39.243) ccw
  line L975 (26.5671, 40.4241) -> (27.2855, 40.4241)
  line L976 (35.3441, 41.2945) -> (36.2145, 40.4241)
  arc A2952 (14.9663, 35.7266) -> (15.2597, 35.8481) centre (15.113, 35.7874) ccw
  line L977 (36.2145, 40.4241) -> (37.4455, 40.4241)
  arc A2953 (12.1897, 39.1812) -> (11.9652, 38.9567) centre (12.0775, 39.069) ccw
  arc A2954 (38.2036, 42.4132) -> (38.4282, 42.6377) centre (38.3159, 42.5255) ccw
  arc A2955 (12.0167, 38.9223) -> (12.1382, 39.2157) centre (12.0775, 39.069) ccw
  arc A2956 (26.5671, 40.5829) -> (26.5671, 40.2654) centre (26.5671, 40.4241) ccw
  arc A2957 (36.3268, 43.2836) -> (36.1023, 43.5082) centre (36.2145, 43.3959) ccw
  arc A2958 (36.2145, 40.5829) -> (36.2145, 40.2654) centre (36.2145, 40.4241) ccw
  arc A2959 (15.2253, 35.2311) -> (15.0007, 35.0066) centre (15.113, 35.1189) ccw
  line L978 (15.6337, 34.2399) -> (15.3804, 34.8514)
  arc A2960 (15.2682, 34.7392) -> (15.4927, 34.9637) centre (15.3805, 34.8514) ccw
  arc A2961 (37.5577, 43.5082) -> (37.3332, 43.2836) centre (37.4455, 43.3959) ccw
  arc A2962 (4.8214, 43.6691) -> (5.1147, 43.5476) centre (4.968, 43.6084) ccw
  arc A2963 (14.9542, 35.1188) -> (15.2717, 35.1188) centre (15.113, 35.1188) ccw
  line L979 (5.1943, 44.7456) -> (4.9681, 45.2917)
  line L980 (0.9017, 44.1544) -> (1.1279, 43.6083)
  arc A2964 (4.4378, 43.3026) -> (4.6623, 43.0781) centre (4.55, 43.1903) ccw
  arc A2965 (0.9812, 43.5476) -> (1.2746, 43.6691) centre (1.1279, 43.6084) ccw
  line L981 (5.1943, 42.2056) -> (4.9681, 42.7517)
  arc A2966 (1.0157, 45.4039) -> (1.2402, 45.1794) centre (1.128, 45.2917) ccw
  arc A2967 (0.755, 44.8063) -> (1.0484, 44.6848) centre (0.9017, 44.7456) ccw
  arc A2968 (4.2037, 40.6787) -> (4.3252, 40.3853) centre (4.2645, 40.532) ccw
  arc A2969 (5.341, 41.5537) -> (5.0476, 41.6752) centre (5.1943, 41.6145) ccw
  line L982 (4.9681, 42.7517) -> (4.5501, 43.1697)
  line L983 (1.5459, 45.7097) -> (1.1279, 45.2917)
  line L984 (1.5459, 43.1903) -> (1.5708, 43.18)
  arc A2970 (1.6582, 45.5974) -> (1.4336, 45.8219) centre (1.5459, 45.7097) ccw
  arc A2971 (4.0647, 46.0826) -> (3.9432, 45.7892) centre (4.004, 45.9359) ccw
  line L985 (4.9681, 45.2917) -> (4.5501, 45.7097)
  arc A2972 (1.2402, 43.7206) -> (1.0157, 43.496) centre (1.1279, 43.6083) ccw
  arc A2973 (0.7429, 44.1544) -> (1.0605, 44.1544) centre (0.9017, 44.1544) ccw
  arc A2974 (5.0803, 40.956) -> (4.8558, 41.1806) centre (4.9681, 41.0683) ccw
  line L986 (4.5501, 43.1903) -> (4.9681, 43.6083)
  line L987 (1.1279, 43.6083) -> (1.5459, 43.1903)
  line L988 (5.1943, 41.6144) -> (5.1943, 42.2056)
  arc A2975 (5.0355, 41.6144) -> (5.353, 41.6144) centre (5.1943, 41.6144) ccw
  arc A2976 (4.6108, 43.0436) -> (4.4894, 43.337) centre (4.5501, 43.1903) ccw
  line L989 (2.092, 45.9359) -> (1.5459, 45.7097)
  arc A2977 (5.341, 44.0937) -> (5.0476, 44.2152) centre (5.1943, 44.1544) ccw
  arc A2978 (4.4893, 45.563) -> (4.6108, 45.8563) centre (4.5501, 45.7097) ccw
  line L990 (4.5501, 43.1697) -> (4.5252, 43.18)
  arc A2979 (2.092, 46.0946) -> (2.092, 45.7771) centre (2.092, 45.9359) ccw
  line L991 (0.9017, 44.7456) -> (0.9017, 44.1544)
  line L992 (1.1279, 45.2917) -> (0.9017, 44.7456)
  arc A2980 (5.0355, 44.1544) -> (5.353, 44.1544) centre (5.1943, 44.1544) ccw
  arc A2981 (4.8558, 45.1794) -> (5.0803, 45.4039) centre (4.9681, 45.2917) ccw
  arc A2982 (4.4644, 43.3267) -> (4.5859, 43.0333) centre (4.5251, 43.18) ccw
  arc A2983 (1.4336, 43.0781) -> (1.6582, 43.3026) centre (1.5459, 43.1904) ccw
  arc A2984 (4.4893, 43.023) -> (4.6108, 43.3163) centre (4.55, 43.1696) ccw
  arc A2985 (1.0605, 44.7456) -> (0.7429, 44.7456) centre (0.9017, 44.7456) ccw
  line L993 (4.5501, 45.7097) -> (4.004, 45.9359)
  arc A2986 (5.353, 42.2056) -> (5.0355, 42.2056) centre (5.1943, 42.2056) ccw
  arc A2987 (1.0484, 44.2152) -> (0.755, 44.0937) centre (0.9017, 44.1544) ccw
  line L994 (4.9681, 41.0683) -> (5.1943, 41.6144)
  arc A2988 (5.1147, 42.8124) -> (4.8214, 42.6909) centre (4.9681, 42.7516) ccw
  arc A2989 (4.8558, 42.6394) -> (5.0803, 42.8639) centre (4.968, 42.7517) ccw
  line L995 (4.5252, 43.18) -> (4.5501, 43.1903)
  arc A2990 (5.0476, 44.6848) -> (5.341, 44.8063) centre (5.1943, 44.7456) ccw
  arc A2991 (4.5859, 43.3267) -> (4.4644, 43.0333) centre (4.5251, 43.18) ccw
  arc A2992 (5.1147, 45.3524) -> (4.8214, 45.2309) centre (4.968, 45.2916) ccw
  arc A2993 (2.1528, 45.7892) -> (2.0313, 46.0826) centre (2.0921, 45.9359) ccw
  arc A2994 (5.353, 44.7456) -> (5.0355, 44.7456) centre (5.1943, 44.7456) ccw
  arc A2995 (4.6108, 40.5036) -> (4.4893, 40.797) centre (4.5501, 40.6503) ccw
  arc A2996 (4.6623, 45.8219) -> (4.4378, 45.5974) centre (4.5501, 45.7097) ccw
  arc A2997 (5.0803, 43.496) -> (4.8558, 43.7206) centre (4.968, 43.6083) ccw
  arc A2998 (5.0476, 42.1448) -> (5.341, 42.2663) centre (5.1943, 42.2056) ccw
  line L996 (5.1943, 44.1544) -> (5.1943, 44.7456)
  arc A2999 (4.8214, 41.1291) -> (5.1147, 41.0076) centre (4.9681, 41.0684) ccw
  line L997 (4.2644, 40.532) -> (4.5501, 40.6503)
  line L998 (4.5501, 40.6503) -> (4.9681, 41.0683)
  arc A3000 (4.004, 45.7771) -> (4.004, 46.0946) centre (4.004, 45.9359) ccw
  arc A3001 (4.6623, 43.2819) -> (4.4378, 43.0574) centre (4.55, 43.1696) ccw
  arc A3002 (1.4852, 45.8563) -> (1.6067, 45.563) centre (1.5459, 45.7097) ccw
  arc A3003 (1.2746, 45.2309) -> (0.9812, 45.3524) centre (1.1279, 45.2917) ccw
  line L999 (4.004, 45.9359) -> (2.092, 45.9359)
  line L1000 (4.9681, 43.6083) -> (5.1943, 44.1544)
  line L1001 (0.9017, 41.6144) -> (1.1279, 41.0683)
  arc A3004 (1.0605, 42.2056) -> (0.7429, 42.2056) centre (0.9017, 42.2056) ccw
  line L1002 (10.9566, 36.957) -> (12.8109, 35.1027)
  arc A3005 (1.9323, 39.4238) -> (2.2257, 39.5453) centre (2.079, 39.4845) ccw
  line L1003 (1.1279, 41.0683) -> (1.5459, 40.6503)
  arc A3006 (1.4851, 43.3163) -> (1.6067, 43.023) centre (1.5459, 43.1696) ccw
  arc A3007 (2.0638, 40.5016) -> (1.7463, 40.5016) centre (1.9051, 40.5016) ccw
  line L1004 (12.8109, 35.1027) -> (12.5596, 34.8514)
  arc A3008 (0.755, 42.2663) -> (1.0484, 42.1448) centre (0.9017, 42.2056) ccw
  arc A3009 (12.4473, 34.9637) -> (12.6718, 34.7392) centre (12.5595, 34.8514) ccw
  arc A3010 (1.6066, 43.337) -> (1.4852, 43.0436) centre (1.5459, 43.1903) ccw
  arc A3011 (4.2233, 37.5648) -> (3.9988, 37.3403) centre (4.111, 37.4526) ccw
  arc A3012 (1.6316, 43.0333) -> (1.5101, 43.3267) centre (1.5708, 43.18) ccw
  arc A3013 (1.6582, 43.0574) -> (1.4336, 43.2819) centre (1.5459, 43.1696) ccw
  line L1005 (4.111, 37.4525) -> (4.4325, 37.131)
  line L1006 (1.905, 39.9046) -> (2.079, 39.4845)
  arc A3014 (1.5101, 43.0333) -> (1.6316, 43.3267) centre (1.5709, 43.18) ccw
  arc A3015 (12.465, 34.2399) -> (12.1476, 34.2399) centre (12.3063, 34.2399) ccw
  arc A3016 (4.7919, 36.8103) -> (4.9134, 37.1037) centre (4.8527, 36.957) ccw
  arc A3017 (4.3203, 37.0188) -> (4.5448, 37.2433) centre (4.4325, 37.1311) ccw
  arc A3018 (1.2402, 41.1806) -> (1.0157, 40.956) centre (1.128, 41.0683) ccw
  arc A3019 (4.4933, 37.2777) -> (4.3718, 36.9843) centre (4.4326, 37.131) ccw
  arc A3020 (1.0157, 42.8639) -> (1.2402, 42.6394) centre (1.128, 42.7517) ccw
  line L1007 (1.5708, 43.18) -> (1.5459, 43.1697)
  arc A3021 (1.0484, 41.6752) -> (0.755, 41.5537) centre (0.9017, 41.6145) ccw
  line L1008 (4.8526, 36.957) -> (10.9566, 36.957)
  line L1009 (1.905, 40.5016) -> (1.905, 39.9046)
  arc A3022 (11.0688, 37.0693) -> (10.8443, 36.8447) centre (10.9566, 36.957) ccw
  arc A3023 (4.4378, 40.7626) -> (4.6623, 40.5381) centre (4.55, 40.6504) ccw
  arc A3024 (1.8442, 40.3549) -> (1.9658, 40.6482) centre (1.905, 40.5016) ccw
  arc A3025 (1.2746, 42.6909) -> (0.9812, 42.8124) centre (1.1279, 42.7516) ccw
  arc A3026 (2.0517, 39.9654) -> (1.7583, 39.8439) centre (1.905, 39.9047) ccw
  arc A3027 (12.1596, 34.3007) -> (12.453, 34.1792) centre (12.3063, 34.24) ccw
  line L1010 (1.5459, 40.6503) -> (1.905, 40.5016)
  arc A3028 (1.4336, 40.5381) -> (1.6582, 40.7626) centre (1.5459, 40.6504) ccw
  arc A3029 (12.9231, 34.9904) -> (12.6986, 35.2149) centre (12.8109, 35.1027) ccw
  line L1011 (0.9017, 42.2056) -> (0.9017, 41.6144)
  line L1012 (12.5596, 34.8514) -> (12.3063, 34.2399)
  line L1013 (1.5459, 43.1697) -> (1.1279, 42.7517)
  line L1014 (2.079, 39.4845) -> (4.111, 37.4525)
  arc A3030 (4.8526, 37.1157) -> (4.8526, 36.7983) centre (4.8526, 36.957) ccw
  line L1015 (4.4325, 37.131) -> (4.8526, 36.957)
  arc A3031 (0.9812, 41.0076) -> (1.2746, 41.1291) centre (1.1279, 41.0684) ccw
  arc A3032 (0.7429, 41.6144) -> (1.0605, 41.6144) centre (0.9017, 41.6144) ccw
  arc A3033 (3.9988, 37.3403) -> (4.2233, 37.5648) centre (4.111, 37.4526) ccw
  arc A3034 (10.9566, 36.7983) -> (10.9566, 37.1157) centre (10.9566, 36.957) ccw
  arc A3035 (1.7463, 39.9046) -> (2.0638, 39.9046) centre (1.9051, 39.9046) ccw
  arc A3036 (1.6067, 40.797) -> (1.4852, 40.5036) centre (1.5459, 40.6503) ccw
  line L1016 (1.1279, 42.7517) -> (0.9017, 42.2056)
  arc A3037 (15.2337, 33.0273) -> (15.5271, 32.9058) centre (15.3804, 32.9666) ccw
  line L1017 (15.3797, 3.81) -> (15.3797, 4.3939)
  arc A3038 (15.7459, 5.5486) -> (15.5214, 5.7731) centre (15.6337, 5.6609) ccw
  arc A3039 (13.8112, 2.4003) -> (14.1287, 2.4003) centre (13.97, 2.4003) ccw
  arc A3040 (12.6986, 34.9904) -> (12.9231, 35.2149) centre (12.8109, 35.1027) ccw
  line L1018 (15.3804, 32.9666) -> (15.6337, 33.5781)
  arc A3041 (13.0883, 32.6452) -> (12.9668, 32.3519) centre (13.0275, 32.4986) ccw
  arc A3042 (13.97, 3.9688) -> (13.97, 3.6513) centre (13.97, 3.81) ccw
  arc A3043 (13.97, 3.9687) -> (13.97, 3.6512) centre (13.97, 3.81) ccw
  line L1019 (14.5539, 2.4003) -> (15.3797, 3.2261)
  arc A3044 (15.3797, 3.6513) -> (15.3797, 3.9688) centre (15.3797, 3.81) ccw
  arc A3045 (15.7804, 33.5173) -> (15.487, 33.6388) centre (15.6337, 33.578) ccw
  arc A3046 (13.6391, 32.404) -> (13.6391, 32.0866) centre (13.6391, 32.2453) ccw
  line L1020 (13.97, 2.4003) -> (13.97, 3.81)
  arc A3047 (12.6718, 33.0788) -> (12.4473, 32.8543) centre (12.5596, 32.9666) ccw
  arc A3048 (15.2209, 3.81) -> (15.5384, 3.81) centre (15.3796, 3.81) ccw
  line L1021 (13.0276, 32.4986) -> (13.6391, 32.2453)
  line L1022 (15.3797, 4.3939) -> (14.8732, 4.9004)
  arc A3049 (15.2674, 4.2817) -> (15.492, 4.5062) centre (15.3797, 4.394) ccw
  arc A3050 (13.97, 3.9687) -> (13.97, 3.6512) centre (13.97, 3.81) ccw
  arc A3051 (15.5384, 4.3939) -> (15.2209, 4.3939) centre (15.3796, 4.3939) ccw
  arc A3052 (2.1913, 39.5968) -> (1.9668, 39.3723) centre (2.0791, 39.4846) ccw
  line L1023 (13.97, 3.81) -> (15.3797, 3.81)
  line L1024 (14.8732, 4.9004) -> (15.6337, 5.6609)
  arc A3053 (14.9732, 32.3519) -> (14.8517, 32.6452) centre (14.9124, 32.4986) ccw
  arc A3054 (12.4129, 32.9058) -> (12.7062, 33.0273) centre (12.5596, 32.9666) ccw
  line L1025 (15.6337, 5.6609) -> (15.6337, 7.0391)
  arc A3055 (13.97, 2.2415) -> (13.97, 2.559) centre (13.97, 2.4003) ccw
  arc A3056 (15.5384, 3.81) -> (15.2209, 3.81) centre (15.3796, 3.81) ccw
  arc A3057 (12.453, 33.6388) -> (12.1596, 33.5173) centre (12.3063, 33.578) ccw
  line L1026 (12.5596, 32.9666) -> (13.0276, 32.4986)
  arc A3058 (13.97, 3.6512) -> (13.97, 3.9687) centre (13.97, 3.81) ccw
  arc A3059 (12.9153, 32.3863) -> (13.1398, 32.6108) centre (13.0275, 32.4986) ccw
  line L1027 (15.3797, 3.2261) -> (15.3797, 3.81)
  line L1028 (13.3861, 2.4003) -> (13.97, 2.4003)
  arc A3060 (10.7132, 8.4483) -> (10.4887, 8.2238) centre (10.601, 8.3361) ccw
  line L1029 (6.2035, 16.2179) -> (5.6955, 16.7259)
  arc A3061 (10.5988, 8.7562) -> (10.3054, 8.6347) centre (10.4521, 8.6955) ccw
  line L1030 (12.3063, 6.6307) -> (12.3063, 5.6609)
  arc A3062 (11.8717, 12.1468) -> (12.0962, 12.3713) centre (11.984, 12.2591) ccw
  arc A3063 (14.1288, 3.81) -> (13.8113, 3.81) centre (13.9701, 3.81) ccw
  line L1031 (14.3009, 32.2453) -> (14.9124, 32.4986)
  arc A3064 (15.2209, 3.2261) -> (15.5384, 3.2261) centre (15.3796, 3.2261) ccw
  line L1032 (4.4645, 13.7541) -> (5.6955, 13.7541)
  line L1033 (12.4079, 9.2951) -> (12.4079, 11.6245)
  arc A3065 (14.8002, 32.6108) -> (15.0247, 32.3863) centre (14.9125, 32.4986) ccw
  line L1034 (7.2149, 14.2621) -> (10.4521, 11.0249)
  arc A3066 (13.97, 2.5591) -> (13.97, 2.2416) centre (13.97, 2.4004) ccw
  arc A3067 (14.761, 5.0126) -> (14.9855, 4.7881) centre (14.8733, 4.9003) ccw
  arc A3068 (14.2402, 32.392) -> (14.3617, 32.0986) centre (14.301, 32.2453) ccw
  line L1035 (13.97, 3.81) -> (13.97, 2.4003)
  arc A3069 (13.3861, 2.559) -> (13.3861, 2.2416) centre (13.3861, 2.4003) ccw
  line L1036 (15.3797, 3.81) -> (13.97, 3.81)
  arc A3070 (13.5783, 32.0986) -> (13.6998, 32.392) centre (13.639, 32.2453) ccw
  arc A3071 (14.1288, 3.81) -> (13.8113, 3.81) centre (13.9701, 3.81) ccw
  arc A3072 (15.4927, 32.8543) -> (15.2682, 33.0788) centre (15.3804, 32.9666) ccw
  arc A3073 (4.4645, 13.9129) -> (4.4645, 13.5954) centre (4.4645, 13.7542) ccw
  arc A3074 (12.0962, 12.3713) -> (11.8717, 12.1468) centre (11.984, 12.2591) ccw
  arc A3075 (15.4749, 5.6609) -> (15.7924, 5.6609) centre (15.6337, 5.6609) ccw
  arc A3076 (8.2862, 16.1813) -> (8.0617, 15.9568) centre (8.1739, 16.0691) ccw
  arc A3077 (7.3272, 14.3744) -> (7.1027, 14.1498) centre (7.2149, 14.2621) ccw
  arc A3078 (15.492, 3.1138) -> (15.2674, 3.3383) centre (15.3797, 3.2261) ccw
  line L1037 (13.97, 2.4003) -> (14.5539, 2.4003)
  arc A3079 (14.9855, 5.0126) -> (14.761, 4.7881) centre (14.8733, 4.9003) ccw
  arc A3080 (14.1287, 3.81) -> (13.8112, 3.81) centre (13.97, 3.81) ccw
  line L1038 (14.9124, 32.4986) -> (15.3804, 32.9666)